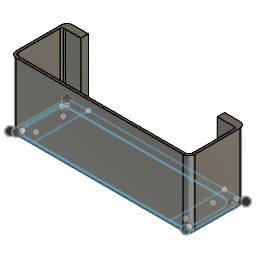
drawer_stop (Autodesk Fusion 360 design; units mm, degrees)
Autodesk Fusion 360 part; units mm, degrees
sketch "Sketch1" plane through (0, 0, 0) normal (0, 0, 1) x (1, 0, 0)
  line L0 (36, 69.573) -> (176.7, 69.573)
  line L1 (181.7, 64.573) -> (181.7, 26.573)
  line L2 (176.7, 21.573) -> (36, 21.573)
  line L3 (31, 26.573) -> (31, 64.573)
  line L4 (49, 23.573) -> (49, 69.5743)
  line L5 (163.7, 69.5743) -> (163.7, 23.573)
  arc A0 (31, 26.573) -> (36, 21.573) centre (36, 26.573) ccw
  arc A1 (36, 69.573) -> (31, 64.573) centre (36, 64.573) ccw
  arc A2 (181.7, 64.573) -> (176.7, 69.573) centre (176.7, 64.573) ccw
  arc A3 (176.7, 21.573) -> (181.7, 26.573) centre (176.7, 26.573) ccw
  line L6 (176.7, 23.573) -> (36, 23.573)
  arc A4 (33, 26.573) -> (36, 23.573) centre (36, 26.573) ccw
  line L7 (33, 26.573) -> (33, 62)
  line L8 (179.7, 61.7919) -> (179.7, 26.573)
  arc A5 (176.7, 23.573) -> (179.7, 26.573) centre (176.7, 26.573) ccw
  line L9 (35.9523, 63.2949) -> (176.6512, 63.292)
  line L10 (176.6512, 63.292) -> (178.2, 63.2919)
  line L11 (33, 62) -> (33, 61.7949)
  line L12 (35.9523, 63.2949) -> (34.5, 63.2949)
  arc A6 (34.5, 63.2949) -> (33, 61.7949) centre (34.5, 61.7949) ccw
  arc A7 (179.7, 61.7919) -> (178.2, 63.2919) centre (178.2, 61.7919) ccw
  line L13 (168.6382, 23.8955) -> (42.6382, 23.8955)
  line L14 (34.6382, 31.8955) -> (34.6382, 54.8955)
  line L15 (42.6382, 62.8955) -> (168.6382, 62.8955)
  line L16 (176.6382, 54.8955) -> (176.6382, 31.8955)
  arc A8 (168.6382, 23.8955) -> (176.6382, 31.8955) centre (168.6382, 31.8955) ccw
  arc A9 (176.6382, 54.8955) -> (168.6382, 62.8955) centre (168.6382, 54.8955) ccw
  arc A10 (34.6382, 31.8955) -> (42.6382, 23.8955) centre (42.6382, 31.8955) ccw
  arc A11 (42.6382, 62.8955) -> (34.6382, 54.8955) centre (42.6382, 54.8955) ccw
  point P0 (31, 69.573)
  point P1 (181.7, 69.573)
  point P2 (31, 21.573)
  point P3 (175.5968, 27.4488)
  point P4 (35.5968, 27.4488)
  point P5 (175.5968, 67.4488)
  point P6 (176.6382, 23.8955)
  point P7 (34.6382, 23.8955)
  point P8 (176.6382, 62.8955)
  dimension "d1" = 150.7
  dimension "d2" = 48
  dimension "d6" = 5
  dimension "d7" = 5
  dimension "d8" = 5
  dimension "d9" = 5
  dimension "d13" = 1.5
  dimension "d14" = 1.5
  dimension "d38" = 140
  dimension "d39" = 40
  dimension "d107" = 142
  dimension "d108" = 39
  dimension "d109" = 8
  constraint horizontal L0
  constraint vertical L1
  constraint horizontal L2
  constraint vertical L3
  constraint coincident L4.start L6
  constraint coincident L5.end L6
  constraint coincident P2 L2
  constraint coincident P2 L3
  constraint tangent L2 A0
  constraint tangent L3 A0
  constraint coincident P0 L0
  constraint coincident P0 L3
  constraint tangent L0 A1
  constraint tangent L3 A1
  constraint coincident P1 L0
  constraint coincident P1 L1
  constraint tangent L0 A2
  constraint tangent L1 A2
  constraint tangent L1 A3
  constraint tangent L2 A3
  constraint parallel L9 L10
  constraint vertical L11
  constraint perpendicular L11 L12
  constraint tangent L12 A6
  constraint tangent L11 A6
  constraint concentric A0 A4
  constraint concentric A3 A5
  constraint tangent L6 A5
  constraint tangent L6 A4
  constraint tangent A4 L7
  constraint tangent L8 A5
  constraint tangent L8 A7
  constraint tangent L10 A7
  constraint horizontal L13
  constraint vertical L14
  constraint horizontal L15
  constraint vertical L16
  constraint coincident P6 L13
  constraint coincident P6 L16
  constraint tangent L13 A8
  constraint tangent L16 A8
  constraint coincident P8 L15
  constraint coincident P8 L16
  constraint tangent L15 A9
  constraint tangent L16 A9
  constraint equal A8 A9
  constraint coincident P7 L13
  constraint coincident P7 L14
  constraint tangent L13 A10
  constraint tangent L14 A10
  constraint equal A8 A10
  constraint tangent L14 A11
  constraint tangent L15 A11
  constraint equal A8 A11
  measures "d1" distance of P0 P1
  measures "d2" distance of P0 P2
  measures "d6" radius of A0
  measures "d7" radius of A1
  measures "d8" radius of A2
  measures "d9" radius of A3
  measures "d13" radius of A6
  measures "d14" radius of A7
  measures "d38" distance of P3 P4
  measures "d39" distance of P3 P5
  measures "d107" distance of P6 P7
  measures "d108" distance of P6 P8
  measures "d109" radius of A8
extrude "Extrude16" add sketch "Sketch1" along normal blind 1.5 contours L4 L5 L9 L15 | L4 L6 A4 L7 L9 L12 A6 L13 L14 L15 A10 A11 | L5 L6 L8 A5 L9 L10 A7 L13 L15 L16 A8 A9 | L4 L5 L6 L13
extrude "Extrude17" add sketch "Sketch1" along normal blind 56 contours L0 L1 L2 L3 L4 L5 A0 A1 A2 A3 L6 A4 L7 L8 A5 L9 L10 L12 A6 A7
extrude "Extrude18" add sketch "Sketch1" along normal blind 6 contours L0 L4 L5 L9
sketch "Sketch7" plane through (0, 69.573, 0) normal (0, 1, 0) x (-1, 0, 0)
  line L0 (-176.7, 0) -> (-36, 0)
  line L1 (-36, 0) -> (-36, 56)
  line L2 (-36, 56) -> (-49, 56)
  line L3 (-49, 56) -> (-49, 6)
  line L4 (-49, 6) -> (-163.7, 6)
  line L5 (-163.7, 6) -> (-163.7, 56)
  line L6 (-163.7, 56) -> (-176.7, 56)
  line L7 (-176.7, 56) -> (-176.7, 0)
  line L8 (-44, 56) -> (-44, 3.5)
  line L9 (-168.7, 3.5) -> (-168.7, 56)
  line L10 (-41.6, 56) -> (-41.6, 0)
  line L11 (-171.1, 0) -> (-171.1, 56)
  line L12 (-171.1, 0) -> (-41.6, 0)
  line L13 (-41.6, 49.5) -> (-44, 49.5)
  line L14 (-168.7, 49.5) -> (-171.1, 49.5)
  line L15 (-168.7, 3.5) -> (-44, 3.5)
  dimension "d116" = -5
  dimension "d117" = -5
  dimension "d118" = -2.4
  dimension "d119" = -2.4
  dimension "d123" = -6.5
  dimension "d124" = -6.5
  dimension "d133" = -3.5
  constraint coincident L11.start L12
  constraint coincident L10.end L12
  constraint coincident L8 L13.end
  constraint coincident L10 L13.start
  constraint coincident L9 L14.start
  constraint coincident L11 L14.end
  constraint coincident L9 L15.start
  constraint perpendicular L9 L15
  constraint coincident L8 L15.end
extrude "Extrude19" add 1 faces at (125.4667, 65.387, 6) along direction (0, 0, 1) blind 3
extrude "Extrude20" cut sketch "Sketch7" against normal blind 4 contours L0 L8 L9 L10 L11 L12 L13 L14 L15
extrude "Extrude21" [rolled back] along distance -5 taper angle 0
